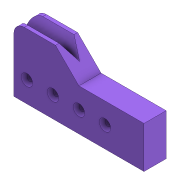
# Autodesk Inventor part: Parameter part
Saved by Autodesk Inventor 2020.1 (Build 241239000, 239)
## iProperties
Created: 2019-10-07
Part Number: Parameter part
Material: Steel
Document SubType Name: Modeling
Designer: thom_tremblay
Density: 7.85 g/cm^3
Appearance: Violet
Author: thom_tremblay
Autodesk Inventor part; units mm, degrees
ref_plane "YZ Plane" through (0, 0, 0) normal (1, 0, 0) x (0, 1, 0)
ref_plane "XZ Plane" through (0, 0, 0) normal (0, 1, 0) x (-1, 0, 0)
ref_plane "XY Plane" through (0, 0, 0) normal (0, 0, 1) x (1, 0, 0)
sketch "Sketch1" plane through (0, 0, 0) normal (0, 0, 1) x (1, 0, 0)
  line L0 (0, 0) -> (127, 0)
  line L1 (127, 0) -> (127, 40.64)
  line L2 (127, 40.64) -> (0, 40.64)
  line L3 (0, 40.64) -> (0, 0)
  line L4 (0, 40.64) -> (0, 53.34)
  arc A0 (10.16, 63.5) -> (0, 53.34) centre (10.16, 53.34) ccw
  line L5 (10.16, 63.5) -> (40.64, 63.5)
  line L6 (40.64, 63.5) -> (63.5, 40.64)
  point P0 (63.5, 0)
  dimension "width" = 127
  dimension "height" = 63.5
  dimension "d2" = 10.16
  dimension "d3" = 45
  dimension "base_height" = 40.64
  constraints: 14 end point, 2 midpoint, 2 parallel, 2 perpendicular, 2 point on circle, 2 tangent, 1 centre point, 1 horizontal, 1 vertical, 1 vertical alignment
  measures "width" distance of L0.start L0.end
  measures "height" distance between parallel lines of L5 L0
  measures "d2" radius of A0
  measures "d3" angle of L2 L6
  measures "base_height" distance of L0.end L1.end
extrude "Extrusion1" add sketch "Sketch1" along normal blind 21.59
sketch "Sketch3" plane through (0, 0, 0) normal (-1, 0, 0) x (0, 0, 1)
  line L0 (18.1273, 63.5) -> (3.4627, 63.5)
  line L1 (3.4627, 63.5) -> (10.795, 50.8)
  line L2 (10.795, 50.8) -> (18.1273, 63.5)
  line L3 (0, 0) -> (21.59, 0) projected
  line L4 (0, 63.5) -> (21.59, 63.5) projected
  point P0 (10.795, 0)
  dimension "d20" = 12.7
  constraints: 6 end point, 2 equal length, 1 horizontal, 1 midpoint, 1 point on line, 1 vertical alignment
  measures "d20" vertical distance of L0.end L1.end
extrude "Extrusion2" cut sketch "Sketch3" against normal through all
sketch "Sketch2" plane through (0, 0, 21.59) normal (0, 0, 1) x (1, 0, 0)
  line L0 (0, 53.34) -> (0, 0) projected
  line L1 (0, 0) -> (127, 0) projected
  point P0 (12.7, 20.32)
  dimension "pat_offset" = 12.7
  dimension "d9" = 20.32
  measures "pat_offset" distance from line of L0 point (12.7, 20.32)
  measures "d9" distance from line of L1 point (12.7, 20.32)
hole "Hole1" at (12.7, 20.32, 21.59) direction (0, 0, -1) diameter 5.7912 end through all countersink diameter 11.1252 countersink angle 82 clearance for "Flat Head Machine Screw (82)" size "#12" standard "Ansi Unified Screw Threads"
pattern_linear "Rectangular Pattern1" count 4 spacing 25.4 along (1, 0, 0) of "Hole1"
equation "\"height\" = 0.5 * width"
equation "\"d9\" = 0.5 * base_height"
body "Solid1"
